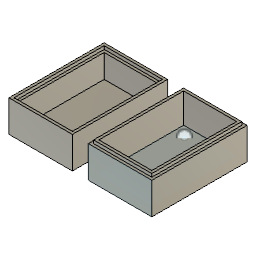
pcb temp case (Autodesk Fusion 360 design; units mm, degrees)
part number: 2025-10-23-15-45-43-296
Autodesk Fusion 360 part; units mm, degrees
sketch "草图1" plane through (0, 0, 0) normal (0, 0, 1) x (1, 0, 0)
  line L0 (0, 0) -> (60, 0)
  line L1 (60, 0) -> (60, -90)
  line L2 (60, -90) -> (0, -90)
  line L3 (0, -90) -> (0, 0)
  dimension "d1" = 60
  dimension "d2" = 90
  constraint horizontal L0
  constraint vertical L1
  constraint horizontal L2
  constraint vertical L3
  constraint coincident L0.start L3.end
  measures "d1" distance of L1 L3
  measures "d2" distance of L0 L2
extrude "拉伸1" add sketch "草图1" along normal blind 30 makes body 1
sketch "草图2" plane through (0, 0, 30) normal (0, 0, 1) x (-1, 0, 0)
  line L0 (0, 90) -> (-60, 90)
  line L1 (-60, 90) -> (-60, 0)
  line L2 (-60, 0) -> (0, 0)
  line L3 (0, 0) -> (0, 90)
  line L4 (-5, 5) -> (-55, 5)
  line L5 (-55, 5) -> (-55, 85)
  line L6 (-55, 85) -> (-5, 85)
  line L7 (-5, 85) -> (-5, 5)
  dimension "d5" = 50
  dimension "d6" = 80
  dimension "d7" = 55
  dimension "d8" = 5
  constraint horizontal L4
  constraint vertical L5
  constraint horizontal L6
  constraint vertical L7
  measures "d5" distance of L5 L7
  measures "d6" distance of L4 L6
  measures "d7" distance of L1 L7
  measures "d8" distance of L2 L4
extrude "拉伸2" cut sketch "草图2" against normal blind 25 contours L4 L5 L6 L7 bodies 1
sketch "草图3" plane through (0, -90, 0) normal (0, -1, 0) x (1, 0, 0)
  line L0 (0, 0) -> (60, 0)
  line L1 (60, 0) -> (60, 30)
  line L2 (60, 30) -> (0, 30)
  line L3 (0, 30) -> (0, 0)
sketch "草图4" plane through (0, 0, 5) normal (0, 0, 1) x (-1, 0, 0)
  line L0 (-5, 85) -> (-55, 85)
  line L1 (-55, 85) -> (-55, 5)
  line L2 (-55, 5) -> (-5, 5)
  line L3 (-5, 5) -> (-5, 85)
  circle A0 centre (-15.0278, 14.2331) radius 0.5
sketch "草图5" plane through (0, 0, 30) normal (0, 0, 1) x (-1, 0, 0)
  line L0 (-55, 5) -> (-55, 85)
  line L1 (-55, 85) -> (-5, 85)
  line L2 (-5, 85) -> (-5, 5)
  line L3 (-5, 5) -> (-55, 5)
  line L4 (0, 90) -> (-60, 90)
  line L5 (-60, 90) -> (-60, 0)
  line L6 (-60, 0) -> (0, 0)
  line L7 (0, 0) -> (0, 90)
  line L8 (-2.5, 2.5) -> (-57.5, 2.5)
  line L9 (-57.5, 2.5) -> (-57.5, 87.5)
  line L10 (-57.5, 87.5) -> (-2.5, 87.5)
  line L11 (-2.5, 87.5) -> (-2.5, 2.5)
  dimension "d12" = 55
  dimension "d13" = 85
  dimension "d14" = 2.5
  dimension "d15" = 87.5
  constraint horizontal L8
  constraint vertical L9
  constraint horizontal L10
  constraint vertical L11
  measures "d12" distance of L9 L11
  measures "d13" distance of L8 L10
  measures "d14" distance of L5 L9
  measures "d15" distance of L6 L10
extrude "拉伸3" add sketch "草图5" along normal blind 3 contours L8 L9 L10 L11 bodies 1
sketch "草图6" plane through (0, 0, 0) normal (0, 0, 1) x (1, 0, 0)
  line L0 (-15, 0) -> (-75, 0)
  line L1 (-75, 0) -> (-75, -90)
  line L2 (-75, -90) -> (-15, -90)
  line L3 (-15, -90) -> (-15, 0)
  dimension "d18" = 60
  dimension "d19" = 90
  dimension "d20" = 15
  constraint horizontal L0
  constraint vertical L1
  constraint horizontal L2
  constraint vertical L3
  constraint horizontal origin L0.start
  measures "d18" distance of L1 L3
  measures "d19" distance of L0 L2
  measures "d20" distance of origin L3
extrude "拉伸4" add sketch "草图6" along normal blind 30 separate body makes body 2
sketch "草图7" plane through (0, 0, 30) normal (0, 0, 1) x (-1, 0, 0)
  line L0 (15, 90) -> (15, 0)
  line L1 (15, 0) -> (75, 0)
  line L2 (75, 0) -> (75, 90)
  line L3 (75, 90) -> (15, 90)
  line L4 (20, 85) -> (70, 85)
  line L5 (70, 85) -> (70, 5)
  line L6 (70, 5) -> (20, 5)
  line L7 (20, 5) -> (20, 85)
  dimension "d23" = 50
  dimension "d24" = 80
  dimension "d25" = 5
  dimension "d26" = 5
  constraint horizontal L4
  constraint vertical L5
  constraint horizontal L6
  constraint vertical L7
  measures "d23" distance of L5 L7
  measures "d24" distance of L4 L6
  measures "d25" distance of L0 L7
  measures "d26" distance of L1 L6
extrude "拉伸5" cut sketch "草图7" against normal blind 25 contours L4 L5 L6 L7 bodies 2
sketch "草图8" plane through (0, 0, 30) normal (0, 0, 1) x (-1, 0, 0)
  line L0 (70, 85) -> (70, 5)
  line L1 (70, 5) -> (20, 5)
  line L2 (20, 5) -> (20, 85)
  line L3 (20, 85) -> (70, 85)
  line L4 (15, 90) -> (15, 0)
  line L5 (15, 0) -> (75, 0)
  line L6 (75, 0) -> (75, 90)
  line L7 (75, 90) -> (15, 90)
  line L8 (17.5, 87.5) -> (72.5, 87.5)
  line L9 (72.5, 87.5) -> (72.5, 2.5)
  line L10 (72.5, 2.5) -> (17.5, 2.5)
  line L11 (17.5, 2.5) -> (17.5, 87.5)
  dimension "d29" = 55
  dimension "d30" = 85
  dimension "d31" = 2.5
  dimension "d32" = 2.5
  constraint horizontal L8
  constraint vertical L9
  constraint horizontal L10
  constraint vertical L11
  measures "d29" distance of L9 L11
  measures "d30" distance of L8 L10
  measures "d31" distance of L4 L11
  measures "d32" distance of L5 L10
extrude "拉伸6" cut sketch "草图8" against normal blind 3 contours L8 L9 L10 L11 bodies 2
